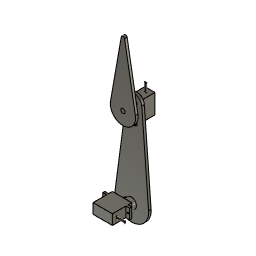
FirstPassArm v8 (Autodesk Fusion 360 design; units mm, degrees)
Autodesk Fusion 360 part; units mm, degrees
sketch "Sketch1" plane through (0, 0, 0) normal (0, 0, 1) x (1, 0, 0) in component "Servo"
  line L0 (0, 0) -> (0, 16)
  line L1 (0, 16) -> (-4.5, 16)
  line L2 (-4.5, 16) -> (-4.5, 18.5)
  line L3 (-4.5, 18.5) -> (0, 18.5)
  line L4 (0, 18.5) -> (0, 23)
  line L5 (0, 23) -> (23, 23)
  line L6 (23, 23) -> (23, 18.5)
  line L7 (23, 18.5) -> (27.5, 18.5)
  line L8 (27.5, 18.5) -> (27.5, 16)
  line L9 (27.5, 16) -> (23, 16)
  line L10 (23, 16) -> (23, 0)
  line L11 (23, 0) -> (0, 0)
  dimension "d1" = 23
  dimension "d2" = 23
  dimension "d3" = 32
  dimension "d4" = 2.5
  dimension "d5" = 16
  constraint coincident L0.start L11.end
  constraint vertical L0
  constraint perpendicular L0 L1
  constraint perpendicular L1 L2
  constraint perpendicular L2 L3
  constraint perpendicular L3 L4
  constraint perpendicular L4 L5
  constraint perpendicular L5 L6
  constraint perpendicular L4 L7
  constraint perpendicular L5 L8
  constraint perpendicular L8 L9
  constraint perpendicular L9 L10
  constraint perpendicular L0 L11
  constraint collinear L1 L9
  constraint equal L7 L9
  constraint equal L3 L7
  constraint equal L1 L3
  constraint collinear L3 L7
  measures "d1" distance of L5 L11
  measures "d2" distance of L10.end L0.start
  measures "d3" distance of L2 L8
  measures "d4" distance of L7.end L8.end
  measures "d5" distance of L9 L11
extrude "Extrude1" add sketch "Sketch1" along normal blind 12 makes body 1 in component "Servo"
sketch "Sketch2" plane through (-0.1121, 23, -0.0426) normal (0, 1, 0) x (-1, 0, 0) in component "Servo"
  line L0 (-23.1121, 0.0426) -> (-0.1121, 0.0426)
  line L1 (-0.1121, 0.0426) -> (-0.1121, 12.0426)
  line L2 (-0.1121, 12.0426) -> (-23.1121, 12.0426)
  line L3 (-23.1121, 12.0426) -> (-23.1121, 0.0426)
  line L4 (-23.1121, 6.0426) -> (-0.1121, 6.0426)
  arc A0 (-11.916, 9.0426) -> (-11.916, 3.0426) centre (-17.1121, 6.0426) ccw
  arc A1 (-11.916, 3.0426) -> (-11.916, 9.0426) centre (-17.1121, 6.0426) ccw construction
  arc A2 (-11.1121, 3.0426) -> (-11.1121, 9.0426) centre (-11.1121, 6.0426) ccw
  line L5 (-11.916, 9.0426) -> (-11.1121, 9.0426)
  line L6 (-11.1121, 3.0426) -> (-11.916, 3.0426)
  dimension "d8" = 6
  dimension "d9" = 3
  constraint midpoint L3 L4.start
  constraint midpoint L1 L4.end
  constraint coincident L4 A0.centre
  constraint vertical A0.start A0.end
  constraint tangent L3 A0
  constraint coincident A0.centre A1.centre
  constraint midpoint A1 A2.centre
  constraint vertical A2.centre A2.start
  constraint vertical A2.start A2.end
  constraint horizontal A0.start A2.end
  measures "d8" radius of A0
  measures "d9" radius of A2
extrude "Extrude2" add sketch "Sketch2" along normal blind 5.5 contours L4 A0 A2 L6 | L4 A0 A2 L5 bodies 1 in component "Servo"
sketch "Sketch3" plane through (0, 28.5, 0) normal (0, 1, 0) x (-1, 0, 0) in component "Servo"
  arc A0 (-11.8038, 9) -> (-11.8038, 3) centre (-17, 6) ccw
  line L0 (-11.8038, 3) -> (-11, 3)
  arc A1 (-11, 3) -> (-11, 9) centre (-11, 6) ccw
  line L1 (-11, 9) -> (-11.8038, 9)
  circle A2 centre (-17, 6) radius 2.5
  dimension "d12" = 5
  constraint concentric A0 A2
  measures "d12" diameter of A2
extrude "Extrude3" add sketch "Sketch3" along normal blind 3.5 contours A2 bodies 1 in component "Servo"
sketch "Sketch4" plane through (23, 0, 0) normal (1, 0, 0) x (0, 1, 0) in component "Servo"
  line L0 (0, 0) -> (16, 0)
  line L1 (16, 0) -> (16, 12)
  line L2 (16, 12) -> (0, 12)
  line L3 (0, 12) -> (0, 0)
  line L4 (5, 12) -> (5, 0) construction
  circle A0 centre (5, 6) radius 0.5
  circle A1 centre (5, 7) radius 0.5
  circle A2 centre (5, 5) radius 0.5
  dimension "d15" = 5
  dimension "d16" = 1
  constraint coincident L2 L4.start
  constraint perpendicular L2 L4
  constraint midpoint L4 A0.centre
  constraint coincident L4 A1.centre
  constraint tangent A0 A1
  constraint coincident L4 A2.centre
  constraint tangent A0 A2
  constraint equal A0 A1
  constraint equal A0 A2
  constraint coincident L0 L4.end
  measures "d15" distance of L3 L4
  measures "d16" diameter of A1
extrude "Extrude4" add sketch "Sketch4" along normal blind 10 separate body contours A0 | A2 | A1 makes body 2 at (26.3333, 5.3749, 5.6692) in component "Servo"
sketch "Sketch5" plane through (0, 18.5, 0) normal (0, 1, 0) x (-1, 0, 0) in component "Servo"
  line L0 (-27.5, 0) -> (-23, 0)
  line L1 (-23, 0) -> (-23, 12)
  line L2 (-23, 12) -> (-27.5, 12)
  line L3 (-27.5, 12) -> (-27.5, 0)
  line L4 (-23, 12) -> (0, 12) construction
  line L5 (-11.5, 12) -> (-11.5, 0) construction
  line L6 (0, 0) -> (0, 12)
  line L7 (0, 0) -> (-17, 0)
  line L8 (-25.5, 6) -> (2.5, 6) construction
  circle A0 centre (2.5, 6) radius 1
  circle A1 centre (-25.5, 6) radius 1
  dimension "d19" = 28
  dimension "d20" = 2
  constraint coincident L1.end L2.start
  constraint perpendicular L1 L4
  constraint midpoint L4 L5.start
  constraint perpendicular L4 L5
  constraint coincident L4.end L6
  constraint coincident L5.end L7
  constraint perpendicular L6 L8
  constraint midpoint L5 L8
  constraint coincident L8.end A0.centre
  constraint coincident L8.start A1.centre
  constraint equal A0 A1
  measures "d19" distance of L8.start L8.end
  measures "d20" diameter of A0
extrude "Extrude5" cut sketch "Sketch5" against normal up to surface (2.5 mm away) contours A0 | A1 bodies 1 in component "Servo"
sketch "Sketch1 (2)" plane through (0, 32, 0) normal (0, 1, 0) x (-1, 0, 0) in component "ArmA"
  circle A0 centre (-17, 6) radius 2.5
  arc A1 (-36.9401, 7.5473) -> (2.8226, 8.6578) centre (-17, 6) ccw
  line L0 (-17, 86) -> (-17, 114) construction
  circle A2 centre (-17, 114) radius 1
  circle A3 centre (-17, 86) radius 1
  line L1 (-17, 100) -> (-23, 100) construction
  line L2 (-23, 111.75) -> (-23, 88.25)
  line L3 (-23, 111.75) -> (-11, 111.75)
  line L4 (-23, 88.25) -> (-7.8491, 88.25)
  line L5 (2.8226, 8.6578) -> (-7.8491, 88.25)
  circle A4 centre (-17, 6) radius 2.5
  line L6 (-36.9401, 7.5473) -> (-28.8932, 111.2502)
  line L7 (-7.8491, 88.25) -> (-11, 111.75) construction
  circle A5 centre (-17, 106) radius 2.5 construction
  arc A6 (-11, 111.75) -> (-28.8932, 111.2502) centre (-19.9202, 110.554) ccw
  circle A7 centre (-17, 6) radius 2.5
  dimension "d38" = 20
  dimension "d39" = 2
  dimension "d40" = 6
  dimension "d41" = 5
  dimension "d43" = 12
  dimension "d44" = 23.5
  dimension "d45" = 5
  dimension "d46" = 8
  dimension "d47" = 28
  dimension "d48" = 100
  dimension "d49" = 9
  constraint coincident A0.centre A1.centre
  constraint vertical L0
  constraint coincident L0.end A2.centre
  constraint coincident L0.start A3.centre
  constraint equal A2 A3
  constraint midpoint L0 L1.start
  constraint perpendicular L0 L1
  constraint perpendicular L1 L2
  constraint midpoint L1.end L2
  constraint perpendicular L0 L3
  constraint perpendicular L2 L4
  constraint concentric A0 A4
  constraint tangent A1 L6
  constraint tangent A1 L5
  constraint parallel L5 L7
  constraint vertical L0.start A0.centre
  constraint coincident L0 A5.centre
  constraint tangent L6 A6
  constraint tangent L7 A6
  measures "d38" radius of A1
  measures "d39" diameter of A2
  measures "d40" distance of L0 L2
  measures "d41" diameter of A4
  measures "d43" distance of L2.start L3.end
  measures "d44" distance of L2.start L2.end
  measures "d45" diameter of A5
  measures "d46" distance of L0.end A5.centre
  measures "d47" distance of L0.start L0.end
  measures "d48" distance of A0.centre A5.centre
  measures "d49" radius of A6
extrude "Extrude1'" add sketch "Sketch1 (2)" against normal blind 3 separate body makes body 3 in component "ArmA"
sketch "Sketch1 (3)" plane through (0, 0, 0) normal (0, 1, 0) x (1, 0, 0) in component "ArmB"
  arc A0 (14.7729, -2.6) -> (-14.7729, -2.6) centre (0, 0) ccw
  circle A1 centre (0, 0) radius 2.5
  line L0 (-14.7729, -2.6) -> (-1.9697, -75.3467)
  line L1 (14.7729, -2.6) -> (1.9697, -75.3467)
  arc A2 (-1.9697, -75.3467) -> (1.9697, -75.3467) centre (0, -75) ccw
  dimension "d60" = 15
  dimension "d61" = 5
  dimension "d62" = 2
  dimension "d63" = 75
  constraint concentric A0 A1
  constraint tangent L0 A2
  constraint tangent L1 A2
  constraint tangent A0 L1
  constraint tangent A0 L0
  constraint horizontal A0.start A0.end
  constraint coincident A0.centre A1.centre
  measures "d60" radius of A0
  measures "d61" diameter of A1
  measures "d62" radius of A2
  measures "d63" distance of A0.centre A2.centre
extrude "Extrude1''" add sketch "Sketch1 (3)" along normal blind 3 separate body makes body 4 in component "ArmB"
component "Servo" placed x (1, 0, 0) y (0, 1, 0) z (0, 0, 1) at (-0.4006, -0.2813, -1.6044)
component "ArmA" placed x (1, 0, 0) y (0, 1, 0) z (0, 0, 1) at (-0.4006, -0.2813, -1.6044)
component "Servo" placed x (0, 0, 1) y (0, -1, 0) z (1, 0, 0) at (10.5994, 50.2187, 86.8956)
component "ArmB" placed x (1, 0, 0) y (0, 1, 0) z (0, 0, 1) at (16.5994, 18.2187, 103.8956)
